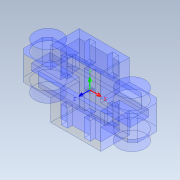
# Autodesk Inventor part: body_inventor
Saved by Autodesk Inventor 2020 (Build 240168000, 168)
## iProperties
Created: 2021-01-07
Part Number: body_inventor
Material: Generic
Document SubType Name: Modeling
Designer: DELL
Density: 1 g/cm^3
Appearance: Clear - Blue
Author: DELL
Autodesk Inventor part; units mm, degrees
ref_plane "YZ Plane" through (0, 0, 0) normal (1, 0, 0) x (0, 1, 0)
ref_plane "XZ Plane" through (0, 0, 0) normal (0, 1, 0) x (-1, 0, 0)
ref_plane "XY Plane" through (0, 0, 0) normal (0, 0, 1) x (1, 0, 0)
sketch "Sketch4" plane through (0, 0, 0) normal (0, 0, 1) x (1, 0, 0)
  line L0 (75, -100) -> (-75, -100)
  line L1 (-75, -100) -> (-75, 100)
  line L2 (-75, 100) -> (75, 100)
  line L3 (75, 100) -> (75, -100)
  line L4 (75, -100) -> (-75, 100) construction
  line L5 (-75, -100) -> (75, 100) construction
  line L6 (170, -37) -> (-170, -37)
  line L7 (-170, -37) -> (-170, 37)
  line L8 (-170, 37) -> (170, 37)
  line L9 (170, 37) -> (170, -37)
  line L10 (170, -37) -> (-170, 37) construction
  line L11 (-170, -37) -> (170, 37) construction
  line L12 (170, 0) -> (-170, 0) construction
  line L13 (25, 90) -> (43, 90)
  line L14 (43, 90) -> (43, -90)
  line L15 (43, -90) -> (25, -90)
  line L16 (25, -90) -> (25, 90)
  line L17 (25, 90) -> (43, -90) construction
  line L18 (43, 90) -> (25, -90) construction
  line L19 (-43, 90) -> (-25, 90)
  line L20 (-25, 90) -> (-25, -90)
  line L21 (-25, -90) -> (-43, -90)
  line L22 (-43, -90) -> (-43, 90)
  line L23 (-43, 90) -> (-25, -90) construction
  line L24 (-25, 90) -> (-43, -90) construction
  line L25 (43, -15) -> (25, -15)
  line L26 (-25, -15) -> (-43, -15)
  line L27 (43, 15) -> (25, 15)
  line L28 (-25, 15) -> (-43, 15)
  line L29 (0, -100) -> (0, 100) construction
  point P0 (0, 0)
  point P1 (0, 0)
  point P2 (0, 0)
  point P3 (75, 37)
  point P4 (-75, 37)
  point P5 (-75, -37)
  point P6 (75, -37)
  point P7 (34, 0)
  point P8 (-34, 0)
  point P9 (43, -37)
  point P10 (25, -37)
  point P11 (-25, -37)
  point P12 (-43, -37)
  point P13 (-43, 37)
  point P14 (-25, 37)
  point P15 (25, 37)
  point P16 (43, 37)
  dimension "d17" = 74
  dimension "d18" = 340
  dimension "d19" = 150
  dimension "d20" = 200
  dimension "d57" = 18
  dimension "d58" = 180
  dimension "d59" = 75
  dimension "d60" = 86
  constraints: 60 end point, 14 point on line, 13 midpoint, 8 parallel, 6 perpendicular, 4 horizontal, 2 collinear, 1 coincident, 2 other
  measures "d17" distance of L8.end L6.start
  measures "d18" distance of L6.start L6.end
  measures "d19" distance of L0.start L0.end
  measures "d20" distance of L2.end L0.start
  measures "d57" distance between parallel lines of L16 L14
  measures "d58" distance of L13.end L14.end
  measures "d59" distance between parallel lines of L15 L25
  measures "d60" distance between parallel lines of L22 L14
extrude "Extrusion4" add sketch "Sketch4" along normal mid plane 85
sketch "Sketch5" plane through (0, 0, 0) normal (0, 1, 0) x (-1, 0, 0)
  circle A0 centre (-125, 0) radius 39.5
  circle A1 centre (125, 0) radius 39.5
  line L0 (75, 42.5) -> (-75, 42.5) construction
  line L1 (0, 42.5) -> (0, -42.5) construction
  line L2 (-75, -42.5) -> (75, -42.5) construction
  line L3 (-170, 42.5) -> (-170, -42.5) construction
  line L4 (-170, 0) -> (170, 0) construction
  line L5 (170, -42.5) -> (170, 42.5) construction
  circle A2 centre (-125, 0) radius 31.5
  circle A3 centre (125, 0) radius 31.5
  line L6 (-155, 42.5) -> (-170, 27.5)
  line L7 (-170, -27.5) -> (-155, -42.5)
  line L8 (-170, -42.5) -> (-75, -42.5) projected
  line L9 (170, 42.5) -> (75, 42.5) projected
  line L10 (155, 42.5) -> (170, 27.5)
  line L11 (170, -27.5) -> (155, -42.5)
  line L12 (-75, 42.5) -> (-170, 42.5) projected
  line L13 (75, -42.5) -> (170, -42.5) projected
  line L14 (-170, 42.5) -> (-170, -42.5)
  line L15 (170, 42.5) -> (170, -42.5)
  circle A4 centre (125, 0) radius 25
  circle A5 centre (-125, 0) radius 25
  point P0 (0, 0)
  point P1 (-170, -27.5)
  dimension "d23" = 79
  dimension "d24" = 250
  dimension "d39" = 63
  dimension "d42" = 15
  dimension "d43" = 45
  dimension "d47" = 50
  constraints: 16 end point, 9 point on line, 6 centre point, 5 perpendicular, 4 coincident, 4 midpoint, 3 equal length, 3 equal radius, 1 symmetric about line
  measures "d23" diameter of A0
  measures "d24" distance of A1.centre A0.centre
  measures "d39" diameter of A2
  measures "d42" distance of L3.start L6.end
  measures "d43" angle of L6 L3
  measures "d47" diameter of A4
extrude "Extrusion5" add sketch "Sketch5" against normal blind 32 from surface at -37 contours A0 | A1 | A2 | A3 | A4 | A5
sketch "Sketch6" plane through (0, 0, 0) normal (0, 0, 1) x (1, 0, 0)
  line L0 (147, 10) -> (-147, 10)
  line L1 (-147, 10) -> (-147, -10)
  line L2 (-147, -10) -> (147, -10)
  line L3 (147, -10) -> (147, 10)
  line L4 (147, 10) -> (-147, -10) construction
  line L5 (-147, 10) -> (147, -10) construction
  line L6 (-60, 90) -> (60, 90)
  line L7 (60, 90) -> (60, -90)
  line L8 (60, -90) -> (-60, -90)
  line L9 (-60, -90) -> (-60, 90)
  line L10 (-60, 90) -> (60, -90) construction
  line L11 (60, 90) -> (-60, -90) construction
  line L12 (75, -100) -> (-75, -100) projected
  line L13 (-75, 37) -> (-75, 100) projected
  line L14 (-170, -37) -> (-170, 37) projected
  line L15 (-75, -37) -> (-170, -37) projected
  point P0 (0, 0)
  point P1 (-60, -10)
  point P2 (60, -10)
  point P3 (60, 10)
  point P4 (-60, 10)
  dimension "d28" = 15
  dimension "d29" = 23
  dimension "d30" = 27
  dimension "d46" = 20
  dimension "d63" = 10
  constraints: 24 end point, 4 midpoint, 4 parallel, 2 horizontal, 2 perpendicular
  measures "d28" distance between parallel lines of L13 L9
  measures "d29" distance between parallel lines of L14 L1
  measures "d30" distance between parallel lines of L15 L2
  measures "d46" distance between parallel lines of L2 L0
  measures "d63" distance between parallel lines of L12 L8
extrude "Extrusion6" cut sketch "Sketch6" along normal mid plane 55
extrude "Extrusion8" cut sketch "Sketch5" against normal through all both and the other way through all contours L6 L14 L12 | L7 L8 L14 | L15 L10 L9 | L15 L13 L11
extrude "Extrusion9" [suppressed]
extrude "Extrusion10" [suppressed]
mirror "Mirror1" about plane through (0, 0, 0) normal (0, 1, 0) of "Extrusion5"
sketch "Sketch7" plane through (0, 0, 0) normal (0, 1, 0) x (-1, 0, 0)
  line L0 (155, -42.5) -> (75, -42.5) projected
  line L1 (110, -42.5) -> (98, -54.5)
  line L2 (98, -54.5) -> (0, -54.5)
  line L3 (75, -42.5) -> (-75, -42.5) projected
  line L4 (0, 0) -> (0, -54.5) construction
  line L5 (0, 0) -> (170, 0) construction
  line L6 (170, -27.5) -> (170, 27.5) construction
  line L7 (-110, -42.5) -> (-98, -54.5)
  line L8 (-98, -54.5) -> (0, -54.5)
  line L9 (-75, -42.5) -> (75, -42.5)
  line L10 (110, 42.5) -> (98, 54.5)
  line L11 (98, 54.5) -> (0, 54.5)
  line L12 (-98, 54.5) -> (0, 54.5)
  line L13 (-110, 42.5) -> (-98, 54.5)
  line L14 (110, -42.5) -> (-110, -42.5)
  line L15 (110, 42.5) -> (-110, 42.5)
  line L16 (155, 42.5) -> (75, 42.5) projected
  point P0 (-75, -42.5)
  dimension "d52" = 12
  dimension "d53" = 45
  dimension "d54" = 98
  constraints: 26 end point, 9 symmetric about line, 2 collinear, 1 midpoint, 1 parallel, 1 point on line, 1 vertical
  measures "d52" distance between parallel lines of L3 L2
  measures "d53" angle of L0 L1
  measures "d54" distance of L1.end L2.end
extrude "Extrusion11" add sketch "Sketch7" along normal mid plane 30
extrude "Extrusion12" cut sketch "Sketch4" along normal through all both and the other way through all contours L14 L15 L16 L6 | L6 L20 L21 L22 | L8 L16 L13 L14 | L22 L19 L20 L8
equation "\"d21\" = body_thickness"
equation "\"d28\" = wall_thickness"
equation "\"d31\" = body_thickness - 2 * wall_thickness"
equation "\"wall_thickness\" = 15"
equation "\"body_thickness\" = 85"
body "Solid1"
body "Solid2"
